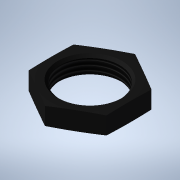
# Autodesk Inventor part: 130519 ESHM-M14x1
Saved by Autodesk Inventor 2021 (Build 250183000, 183)
## iProperties
Created: 2026-04-19
Part Number: 130519 ESHM-M14x1
Material: Generic
Catalog Web Link: www.3dfindit.com
Description: ESHM-Mounting nut
Vendor: FESTO
Document SubType Name: Modeling
Designer: psAdmin
Manufacturer: FESTO
Mass: 0.463106 g
Surface Area: 6.06905 cm^2
Volume: 0.463106 cm^3
Density: 1 g/cm^3
Appearance: PSOLRGB-128-128-128
Category: PARTsolutions
Company: FESTO
Title: 130519 ESHM-M14x1
Author: Cadenas PARTsolutions
Comments: Mounting nut
PSOL_IDENT_0: {$CADENAS_DATA/23d-libs/festo/parts/e/esh/nuts/eshm.prj},172 {VTYP=3D},{NB=130519 ESHM-M14x1},{LINA=
PSOL_IDENT_1: 130519 ESHM-M14x1},{NN=ESHM},{DATE=20.05.2020 09:49:53},{GEOMDATE=02.09.2015 14:27:48},{VERSION=},{L
PSOL_IDENT_2: INEID=60},{WBVAR=},{WBNUMERIC=}  {NB=130519 ESHM-M14x1},{LINA=130519 ESHM-M14x1},{KT=DUMMY},{TNR=130
PSOL_IDENT_3: 519},{TYP=ESHM},{M=M14x1},{MN=14.000},{P=1.000},{SW=17.000},{H=4.000}
NB: 130519 ESHM-M14x1
NN: ESHM
NT: Mounting nut
NBSYN: $TNR. $TYP.-$M.
LINA: 130519 ESHM-M14x1
CATALOG: Festo
TNR: 130519
TYP: ESHM
M: M14x1
MN: 14
P: 1
SW: 17
H: 4
SUPPLIER: FESTO
ARTICLENO: 130519 ESHM-M14x1
BOMINFO: 130519 ESHM-M14x1
CREATOR: CADENAS GmbH
Autodesk Inventor part; units mm, degrees
sketch "Skizze_1" plane through (0, 0, 0) normal (0, 0, 1) x (1, 0, 0)
  line L0 (0, 0) -> (0, 4)
  line L1 (0, 4) -> (8.5, 4)
  line L2 (8.5, 4) -> (12.75, 3.6282)
  line L3 (12.75, 3.6282) -> (12.75, 0.3718)
  line L4 (12.75, 0.3718) -> (8.5, 0)
  line L5 (8.5, 0) -> (0, 0)
  line L6 (0, 0) -> (0, 4)
  constraints: 14 end point
revolve "Revolution1" add sketch "Skizze_1" angle 360 about axis through (0, 0, 0) along (0, -1, 0)
sketch "Skizze_2" plane through (0, 4, 0) normal (0, 1, 0) x (1, 0, 0)
  line L0 (-17, 17) -> (-17, -17)
  line L1 (-17, -17) -> (17, -17)
  line L2 (17, -17) -> (17, 17)
  line L3 (17, 17) -> (-17, 17)
  line L4 (-8.5, -4.9075) -> (0, -9.815)
  line L5 (0, -9.815) -> (8.5, -4.9075)
  line L6 (8.5, -4.9075) -> (8.5, 4.9075)
  line L7 (8.5, 4.9075) -> (0, 9.815)
  line L8 (0, 9.815) -> (-8.5, 4.9075)
  line L9 (-8.5, 4.9075) -> (-8.5, -4.9075)
  constraints: 20 end point
extrude "Extrusion1" cut sketch "Skizze_2" along normal mid plane 8
sketch "Sketch_1" plane through (0, 0, 0) normal (0, 0, 1) x (1, 0, 0)
  line L0 (0, 0) -> (0, 4)
  line L1 (0, 4) -> (7, 4)
  line L2 (7, 4) -> (6.4585, 3.4585)
  line L3 (6.4585, 3.4585) -> (6.4585, 0.5415)
  line L4 (6.4585, 0.5415) -> (7, 0)
  line L5 (7, 0) -> (0, 0)
  line L6 (0, 0) -> (0, 4)
  constraints: 14 end point
revolve "Revolution2" cut sketch "Sketch_1" angle 360 about axis through (0, 0, 0) along (0, -1, 0)
thread "Thread1" size "M14x1" class "6H" standard "ISO Metric profile" full length
ref_plane "ANBAU_XY" through (0, 0, 0) normal (0, 1, 0) x (1, 0, 0)
ref_plane "ANBAU_YZ" through (0, 0, 0) normal (1, 0, 0) x (0, 0, -1)
ref_plane "ANBAU_ZX" through (0, 0, 0) normal (0, 0, -1) x (0, 1, 0)
body "Solid1"
